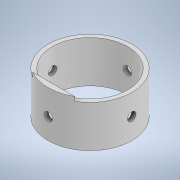
# Autodesk Inventor part: aiirframe
Saved by Autodesk Inventor 2022 (Build 260153000, 153)
## iProperties
Created: 2021-09-22
Part Number: aiirframe
Material: Generic
Document SubType Name: Modeling
Designer: WASHINGTON
Density: 1 g/cm^3
Appearance: Default
Author: WASHINGTON
Autodesk Inventor part; units mm, degrees
ref_plane "YZ Plane" through (0, 0, 0) normal (1, 0, 0) x (0, 1, 0)
ref_plane "XZ Plane" through (0, 0, 0) normal (0, 1, 0) x (-1, 0, 0)
ref_plane "XY Plane" through (0, 0, 0) normal (0, 0, 1) x (1, 0, 0)
sketch "Sketch1" plane through (0, 0, 0) normal (0, 1, 0) x (-1, 0, 0)
  circle A0 centre (0, 0) radius 45
  circle A1 centre (0, 0) radius 50
  dimension "d0" = 90
  dimension "d1" = 100
  constraints: 2 centre point, 2 coincident
  measures "d0" diameter of A0
  measures "d1" diameter of A1
sketch "Sketch1 outline for Extrusion1" plane through (0, 0, 0) normal (0, 1, 0) x (-1, 0, 0)
  circle A0 centre (0, 0) radius 50
  circle A1 centre (0, 0) radius 45
extrude "Extrusion1" add sketch "Sketch1 outline for Extrusion1" along normal mid plane 50
sketch "Sketch2" plane through (0, 25, 0) normal (0, 1, 0) x (1, 0, 0)
  circle A0 centre (0, 0) radius 50
  line L0 (-25, -43.30127) -> (-22.923274, -43.30127)
  line L1 (-25, -43.30127) -> (25, -43.30127)
  line L2 (-22.923274, -43.30127) -> (-25, -43.30127)
  arc A1 (-25, -43.30127) -> (25, -43.30127) centre (0, 0) ccw
  dimension "d16" = 25
  constraints: 6 end point, 4 point on circle, 1 centre point, 1 coincident, 1 horizontal
  measures "d16" horizontal distance of point (0, 0) L1.end
sketch "Sketch2 outline for Extrusion2" plane through (0, 25, 0) normal (0, 1, 0) x (1, 0, 0)
  line L0 (25, -43.30127) -> (-22.923274, -43.30127)
  arc A0 (-25, -43.30127) -> (25, -43.30127) centre (0, 0) ccw
  line L1 (-22.923274, -43.30127) -> (-25, -43.30127)
extrude "Extrusion2" add sketch "Sketch2 outline for Extrusion2" along normal blind 5
sketch "Sketch3" plane through (0, 0, 0) normal (0, 0, 1) x (1, 0, 0)
  circle A0 centre (0, 0) radius 5
  dimension "d10" = 10
  constraints: 1 centre point, 1 coincident
  measures "d10" diameter of A0
sketch "Sketch3 outline for Extrusion3" plane through (0, 0, 0) normal (0, 0, 1) x (1, 0, 0)
  circle A0 centre (0, 0) radius 5
extrude "Extrusion3" cut sketch "Sketch3 outline for Extrusion3" along normal through all both and the other way through all
sketch "Sketch4" plane through (0, 0, 0) normal (1, 0, 0) x (0, 1, 0)
  circle A0 centre (0, 0) radius 5
  dimension "d13" = 10
  constraints: 1 centre point, 1 coincident
  measures "d13" diameter of A0
sketch "Sketch4 outline for Extrusion4" plane through (0, 0, 0) normal (1, 0, 0) x (0, 1, 0)
  circle A0 centre (0, 0) radius 5
extrude "Extrusion4" cut sketch "Sketch4 outline for Extrusion4" along normal through all both and the other way through all
body "Solid1"
